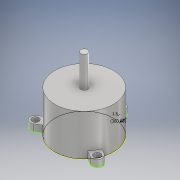
# Autodesk Inventor part: motor_design2
Saved by Autodesk Inventor 2017 (Build 210142000, 142)
## iProperties
Created: 2018-04-04
Part Number: motor_design2
Material: Aluminum 6061-AHC
Document SubType Name: Modeling
Designer: Roland
Density: 2.7 g/cm^3
Appearance: Aluminum - Dark
Author: Roland
Autodesk Inventor part; units mm, degrees
ref_plane "YZ Plane" through (0, 0, 0) normal (1, 0, 0) x (0, 1, 0)
ref_plane "XZ Plane" through (0, 0, 0) normal (0, 1, 0) x (-1, 0, 0)
ref_plane "XY Plane" through (0, 0, 0) normal (0, 0, 1) x (1, 0, 0)
sketch "Sketch1" plane through (0, 0, 0) normal (0, 0, 1) x (1, 0, 0)
  circle A0 centre (0, 0) radius 8.5
  dimension "d0" = 17
  constraints: 1 centre point, 1 coincident
  measures "d0" diameter of A0
extrude "Extrusion1" add sketch "Sketch1" along normal blind 12
sketch "Sketch2" plane through (0, 0, 0) normal (0, 0, -1) x (-1, 0, 0)
  circle A0 centre (0, 0) radius 8.5 projected
  line L0 (-1.5, 8.3666) -> (-1.5, 10.3666)
  line L1 (1.5, 8.3666) -> (1.5, 10.3666)
  arc A1 (1.5, 10.3666) -> (-1.5, 10.3666) centre (0, 10.3666) ccw
  line L2 (-6.4957, -5.4823) -> (-8.2277, -6.4823)
  line L3 (-7.9957, -2.8843) -> (-9.7277, -3.8843)
  arc A2 (-9.7277, -3.8843) -> (-8.2277, -6.4823) centre (-8.9777, -5.1833) ccw
  line L4 (7.9957, -2.8843) -> (9.7277, -3.8843)
  line L5 (6.4957, -5.4823) -> (8.2277, -6.4823)
  arc A3 (8.2277, -6.4823) -> (9.7277, -3.8843) centre (8.9777, -5.1833) ccw
  arc A4 (-7.9957, -2.8843) -> (-6.4957, -5.4823) centre (0, 0) ccw
  arc A5 (6.4957, -5.4823) -> (7.9957, -2.8843) centre (0, 0) ccw
  dimension "d4" = 2
  dimension "d7" = 360
  dimension "d21" = 1.5
  constraints: 12 end point, 12 point on circle, 5 centre point, 3 coincident, 2 tangent, 2 vertical, 1 concentric, 25 other
  measures "d4" distance of L0.start L0.end
  measures "d21" distance from line of L1 A1.centre
extrude "Extrusion2" add sketch "Sketch2" against normal blind 2 contours A0 L0 A1 L1 | L4 A3 L5 A0 | A0 L2 A2 L3
hole "Hole1" at (-8.9777, -5.1833, 0) at (8.9777, -5.1833, 0) at (0, 10.3666, 0) direction (0, 0, 1) diameter 2 end through all
sketch "Sketch3" plane through (0, 0, 12) normal (0, 0, 1) x (1, 0, 0)
  circle A0 centre (0, 0) radius 1
  dimension "d18" = 2
  constraints: 1 centre point, 1 coincident
  measures "d18" diameter of A0
extrude "Extrusion3" add sketch "Sketch3" along normal blind 9
body "Solid1"
